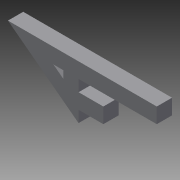
# Autodesk Inventor part: wedger
Saved by Autodesk Inventor 2013 (Build 170138000, 138)
## iProperties
Created: 2013-02-25
Part Number: wedger
Material: Generic
Document SubType Name: Modeling
Designer: Arpan
Density: 1 g/cm^3
Author: Arpan
Autodesk Inventor part; units mm, degrees
ref_plane "YZ Plane" through (0, 0, 0) normal (1, 0, 0) x (0, 1, 0)
ref_plane "XZ Plane" through (0, 0, 0) normal (0, 1, 0) x (-1, 0, 0)
ref_plane "XY Plane" through (0, 0, 0) normal (0, 0, 1) x (1, 0, 0)
sketch "Sketch1" plane through (0, 0, 0) normal (0, 0, 1) x (1, 0, 0)
  line L0 (0, 0) -> (-158.75, 0)
  line L1 (-158.75, 0) -> (-41.275, -88.9)
  line L2 (-41.275, -88.9) -> (-41.275, 0)
  line L3 (-41.275, -88.9) -> (-41.275, -69.85)
  line L4 (-41.275, -69.85) -> (0, -69.85)
  line L5 (0, -69.85) -> (0, 0)
  line L6 (-41.275, 0) -> (-66.675, 0)
  line L7 (-66.675, 0) -> (-66.675, -69.6784)
  line L8 (-66.675, 0) -> (-66.675, -25.4)
  line L9 (-66.675, -25.4) -> (-125.1857, -25.4)
  line L10 (-94.622, -48.5293) -> (-79.2945, -28.2752)
  line L11 (-79.2945, -28.2752) -> (-83.0939, -25.4)
  line L12 (-79.2945, -28.2752) -> (-66.675, -37.8251)
  line L13 (-41.275, -69.85) -> (-41.275, -44.45)
  line L14 (-41.275, -44.45) -> (0, -44.45)
  line L15 (-41.275, 0) -> (-41.275, -25.4)
  line L16 (0, 0) -> (0, -25.4)
  line L17 (-41.275, -25.4) -> (0, -25.4)
  line L18 (0, -25.4) -> (88.9, -25.4)
  line L19 (88.9, -25.4) -> (88.9, 0)
  line L20 (88.9, 0) -> (0, 0)
  dimension "d0" = 158.75
  dimension "d1" = 88.9
  dimension "d2" = 41.275
  dimension "d3" = 19.05
  dimension "d4" = 25.4
  dimension "d5" = 25.4
  dimension "d6" = 25.4
  dimension "d7" = 25.4
  dimension "d8" = 25.4
  dimension "d9" = 88.9
  constraints: 42 end point, 12 point on line, 9 perpendicular, 3 collinear, 1 horizontal, 1 midpoint, 1 parallel
  measures "d0" distance of L0.start L0.end
  measures "d1" distance of L1.end L2.end
  measures "d2" distance from line of L0.start L2
  measures "d3" distance of L1.end L3.end
  measures "d4" distance of L2.end L6.end
  measures "d5" distance of L6.end L8.end
  measures "d6" distance of L10.start L10.end
  measures "d7" distance of L3.end L13.end
  measures "d8" distance of L2.end L15.end
  measures "d9" distance of L16.end L18.end
extrude "Extrusion1" add sketch "Sketch1" along normal blind 25.4 contours L5 L17 L2 L0 | L20 L19 L18 L5 | L2 L1 L7 L0 | L7 L9 L1 L0 | L5 L4 L2 L14 | L9 L11 L10 L1 | L7 L1 L10 L12
body "Solid1"
